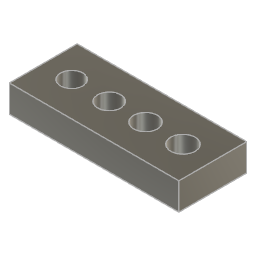
Untitled v1 (Autodesk Fusion 360 design; units mm, degrees)
Autodesk Fusion 360 part; units mm, degrees
sketch "Sketch1" plane through (0, 0, 0) normal (0, 0, 1) x (1, 0, 0)
  line L0 (0, 0) -> (25, 0)
  line L1 (25, 0) -> (25, -10)
  line L2 (25, -10) -> (0, -10)
  line L3 (0, -10) -> (0, 0)
  dimension "d9" = 25
  constraint horizontal L0
  constraint vertical L1
  constraint horizontal L2
  constraint vertical L3
  constraint coincident L0.start L3.end
  measures "d9" distance of L1 L3
extrude "Extrude1" add sketch "Sketch1" along normal blind 4
sketch "Sketch2" plane through (0, 0, 4) normal (0, 0, 1) x (-1, 0, 0)
  line L0 (0, 10) -> (-25, 10)
  line L1 (-25, 10) -> (-25, 0)
  line L2 (-25, 0) -> (0, 0)
  line L3 (0, 0) -> (0, 10)
  circle A0 centre (-4.1436, 4.9511) radius 1.65
  circle A1 centre (-9.7134, 4.9878) radius 1.7
  circle A2 centre (-15.0445, 4.9539) radius 1.75
  circle A3 centre (-20.6276, 5.0224) radius 1.8
  dimension "d3" = 3.3
  dimension "d4" = 3.4
  dimension "d5" = 3.5
  dimension "d6" = 3.6
  measures "d3" diameter of A0
  measures "d4" diameter of A1
  measures "d5" diameter of A2
  measures "d6" diameter of A3
extrude "Extrude2" cut sketch "Sketch2" against normal blind 7 contours A0 | A1 | A2 | A3
